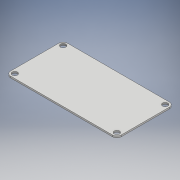
# Autodesk Inventor part: Paneeltje
Saved by Autodesk Inventor 2018 (Build 220112000, 112)
## iProperties
Created: 2018-02-27
Part Number: Paneeltje
Material: Generic
Document SubType Name: Modeling
Designer: Dieter Vansteenwegen
Density: 1 g/cm^3
Appearance: Default
Author: Dieter Vansteenwegen
Autodesk Inventor part; units mm, degrees
ref_plane "YZ Plane" through (0, 0, 0) normal (1, 0, 0) x (0, 1, 0)
ref_plane "XZ Plane" through (0, 0, 0) normal (0, 1, 0) x (-1, 0, 0)
ref_plane "XY Plane" through (0, 0, 0) normal (0, 0, 1) x (1, 0, 0)
sketch "Sketch1" plane through (0, 0, 0) normal (0, 0, 1) x (1, 0, 0)
  line L0 (-47.5, 26.5) -> (47.5, 26.5)
  line L1 (51.5, 22.5) -> (51.5, -22.5)
  line L2 (47.5, -26.5) -> (-47.5, -26.5)
  line L3 (-51.5, -22.5) -> (-51.5, 22.5)
  arc A0 (-51.5, -22.5) -> (-47.5, -26.5) centre (-47.5, -22.5) ccw
  arc A1 (47.5, -26.5) -> (51.5, -22.5) centre (47.5, -22.5) ccw
  arc A2 (51.5, 22.5) -> (47.5, 26.5) centre (47.5, 22.5) ccw
  arc A3 (-47.5, 26.5) -> (-51.5, 22.5) centre (-47.5, 22.5) ccw
  line L4 (-47.51, 22.5) -> (47.51, 22.5) construction
  line L5 (47.51, 22.5) -> (47.51, -22.5) construction
  line L6 (47.51, -22.5) -> (-47.51, -22.5) construction
  line L7 (-47.51, -22.5) -> (-47.51, 22.5) construction
  circle A4 centre (-47.51, 22.5) radius 2.5
  circle A5 centre (47.51, 22.5) radius 2.5
  circle A6 centre (-47.51, -22.5) radius 2.5
  circle A7 centre (47.51, -22.5) radius 2.5
  point P0 (0, 0)
  point P1 (-51.5, 26.5)
  point P2 (51.5, -26.5)
  point P3 (51.5, 26.5)
  point P4 (0, 26.5)
  point P5 (51.5, 0)
  point P6 (47.51, 0)
  point P7 (0, 22.5)
  dimension "d0" = 103
  dimension "d1" = 53
  dimension "d3" = 4
  dimension "d4" = 95.02
  dimension "d5" = 45
  dimension "d6" = 5
  dimension "d7" = 5
  dimension "d8" = 5
  dimension "d9" = 5
  constraints: 16 end point, 8 centre point, 8 point on circle, 8 tangent, 6 point on line, 4 coincident, 4 midpoint, 4 parallel, 3 equal radius, 2 horizontal, 2 horizontal alignment, 2 perpendicular, 2 vertical alignment
  measures "d0" distance of point (-51.5, 26.5) point (51.5, 26.5)
  measures "d1" distance of point (51.5, 26.5) point (51.5, -26.5)
  measures "d3" radius of A0
  measures "d4" distance of L4.start L4.end
  measures "d5" distance of L4.end L5.end
  measures "d6" diameter of A4
  measures "d7" diameter of A5
  measures "d8" diameter of A6
  measures "d9" diameter of A7
extrude "Extrusion1" add sketch "Sketch1" along normal mid plane 1.5
body "Solid1"
